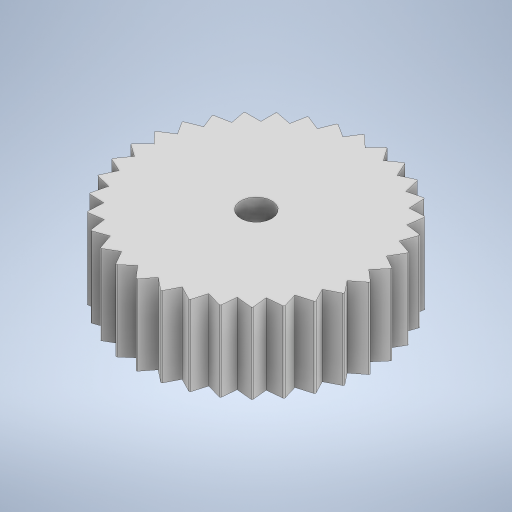
# Autodesk Inventor part: wheel
Saved by Autodesk Inventor 2024 (Build 280153000, 153)
## iProperties
Created: 2024-05-14
Part Number: wheel
Material: Generic
Document SubType Name: Modeling
Designer: david
Density: 1 g/cm^3
Appearance: Default
Author: david
Autodesk Inventor part; units mm, degrees
ref_plane "YZ Plane" through (0, 0, 0) normal (1, 0, 0) x (0, 1, 0)
ref_plane "XZ Plane" through (0, 0, 0) normal (0, 1, 0) x (-1, 0, 0)
ref_plane "XY Plane" through (0, 0, 0) normal (0, 0, 1) x (1, 0, 0)
sketch "Sketch1" plane through (0, 0, 0) normal (0, 1, 0) x (-1, 0, 0)
  circle A0 centre (0, 0) radius 12
  dimension "d0" = 24
  constraints: 1 centre point, 1 coincident
  measures "d0" diameter of A0
extrude "Extrusion1" add sketch "Sketch1" along normal blind 8
sketch "Sketch2" plane through (0, 8, 0) normal (0, 1, 0) x (1, 0, 0)
  circle A0 centre (0, 0) radius 12 projected
  line L0 (0, -12) -> (0.9599, -10.7743)
  line L1 (0.9599, -10.7743) -> (2.2536, -11.7875)
  line L2 (2.271, -11.7831) -> (2.9816, -10.398)
  line L3 (2.9816, -10.398) -> (4.4436, -11.148)
  line L4 (4.4599, -11.1404) -> (4.8955, -9.6458)
  line L5 (4.8955, -9.6458) -> (6.4731, -10.1056)
  line L6 (6.4877, -10.095) -> (6.6325, -8.545)
  line L7 (6.6325, -8.545) -> (8.2686, -8.6979)
  line L8 (8.2809, -8.6848) -> (8.1298, -7.1354)
  line L9 (8.1298, -7.1354) -> (9.7653, -6.9759)
  line L10 (9.7749, -6.9607) -> (9.3333, -5.4679)
  line L11 (9.3333, -5.4679) -> (10.909, -5.0017)
  line L12 (10.9156, -4.985) -> (10.1994, -3.6027)
  line L13 (10.1994, -3.6027) -> (11.6584, -2.8468)
  line L14 (11.6617, -2.8291) -> (10.6969, -1.6074)
  line L15 (10.6969, -1.6074) -> (11.9865, -0.589)
  line L16 (11.9864, -0.571) -> (10.8078, 0.4461)
  line L17 (10.8078, 0.4461) -> (11.8814, 1.6901)
  line L18 (11.8779, 1.7078) -> (10.5281, 2.4834)
  line L19 (10.5281, 2.4834) -> (11.3468, 3.9082)
  line L20 (11.34, 3.9248) -> (9.8678, 4.431)
  line L21 (9.8678, 4.431) -> (10.4021, 5.9849)
  line L22 (10.3923, 6) -> (8.8509, 6.2184)
  line L23 (8.8509, 6.2184) -> (9.0815, 7.8454)
  line L24 (9.069, 7.8583) -> (7.5141, 7.7811)
  line L25 (7.5141, 7.7811) -> (7.4326, 9.4223)
  line L26 (7.4179, 9.4326) -> (5.9058, 9.0625)
  line L27 (5.9058, 9.0625) -> (5.5151, 10.6586)
  line L28 (5.4987, 10.666) -> (4.0839, 10.0164)
  line L29 (4.0839, 10.0164) -> (3.3983, 11.5098)
  line L30 (3.3808, 11.5139) -> (2.1145, 10.6083)
  line L31 (2.1145, 10.6083) -> (1.1586, 11.9449)
  line L32 (1.1407, 11.9457) -> (0.0687, 10.8168)
  line L33 (0.0687, 10.8168) -> (-1.1229, 11.9483)
  line L34 (-1.1407, 11.9457) -> (-1.9797, 10.6343)
  line L35 (-1.9797, 10.6343) -> (-3.3638, 11.5199)
  line L36 (-3.3808, 11.5139) -> (-3.9565, 10.0675)
  line L37 (-3.9565, 10.0675) -> (-5.4832, 10.6751)
  line L38 (-5.4987, 10.666) -> (-5.7902, 9.1368)
  line L39 (-5.7902, 9.1368) -> (-7.4044, 9.4445)
  line L40 (-7.4179, 9.4326) -> (-7.4148, 7.8759)
  line L41 (-7.4148, 7.8759) -> (-9.058, 7.8725)
  line L42 (-9.069, 7.8583) -> (-8.7713, 6.3303)
  line L43 (-8.7713, 6.3303) -> (-10.3842, 6.016)
  line L44 (-10.3923, 6) -> (-9.8108, 4.5559)
  line L45 (-9.8108, 4.5559) -> (-11.335, 3.9421)
  line L46 (-11.34, 3.9248) -> (-10.4957, 2.6169)
  line L47 (-10.4957, 2.6169) -> (-11.8762, 1.7257)
  line L48 (-11.8779, 1.7078) -> (-10.8013, 0.5833)
  line L49 (-10.8013, 0.5833) -> (-11.9882, -0.5531)
  line L50 (-11.9864, -0.571) -> (-10.7165, -1.4714)
  line L51 (-10.7165, -1.4714) -> (-11.6669, -2.8119)
  line L52 (-11.6617, -2.8291) -> (-10.2443, -3.4729)
  line L53 (-10.2443, -3.4729) -> (-10.9239, -4.969)
  line L54 (-10.9156, -4.985) -> (-9.402, -5.3489)
  line L55 (-9.402, -5.3489) -> (-9.7861, -6.9466)
  line L56 (-9.7749, -6.9607) -> (-8.2198, -7.0316)
  line L57 (-8.2198, -7.0316) -> (-8.2946, -8.6731)
  line L58 (-8.2809, -8.6848) -> (-6.7405, -8.4601)
  line L59 (-6.7405, -8.4601) -> (-6.5033, -10.0861)
  line L60 (-6.4877, -10.095) -> (-5.0176, -9.5829)
  line L61 (-5.0176, -9.5829) -> (-4.477, -11.1346)
  line L62 (-4.4599, -11.1404) -> (-3.1133, -10.3593)
  line L63 (-3.1133, -10.3593) -> (-2.2888, -11.7807)
  line L64 (-2.271, -11.7831) -> (-1.0966, -10.7613)
  line L65 (-1.0966, -10.7613) -> (-0.018, -12.001)
  point P0 (-8.2946, -8.6718)
  dimension "d5" = 360
  constraints: 132 end point, 1 perpendicular, 168 other
extrude "Extrusion2" cut sketch "Sketch2" against normal blind 8 contours A0 L56 L57
pattern_circular "Circular Pattern1" count 33 over 360 about axis through (0, -10, 0) along (0, 1, 0) of "Extrusion2"
fillet "Fillet1" radius 0.1 2 edges at (-1.1219, 4, -11.9474) (-1.1407, 4, -11.9457)
pattern_circular "Circular Pattern2" count 33 over 360 about axis through (0, -10, 0) along (0, 1, 0) of "Fillet1"
sketch "Sketch3" plane through (0, 8, 0) normal (0, 1, 0) x (1, 0, 0)
  circle A0 centre (0, 0) radius 1.55
  dimension "d16" = 3.1
  constraints: 1 centre point, 1 coincident
  measures "d16" diameter of A0
extrude "Extrusion3" cut sketch "Sketch3" against normal blind 8
body "Solid1"
